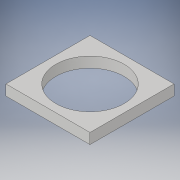
# Autodesk Inventor part: MarbleRingTest3
Saved by Autodesk Inventor 2018 (Build 220112000, 112)
## iProperties
Created: 2019-03-20
Part Number: MarbleRingTest3
Material: Generic
Document SubType Name: Modeling
Designer: 871357
Density: 1 g/cm^3
Appearance: Default
Author: 871357
Autodesk Inventor part; units mm, degrees
ref_plane "YZ Plane" through (0, 0, 0) normal (1, 0, 0) x (0, 1, 0)
ref_plane "XZ Plane" through (0, 0, 0) normal (0, 1, 0) x (-1, 0, 0)
ref_plane "XY Plane" through (0, 0, 0) normal (0, 0, 1) x (1, 0, 0)
sketch "Sketch1" plane through (0, 0, 0) normal (0, 1, 0) x (-1, 0, 0)
  circle A0 centre (0, 0) radius 8.255
  line L0 (10.16, -10.16) -> (-10.16, -10.16)
  line L1 (-10.16, -10.16) -> (-10.16, 10.16)
  line L2 (-10.16, 10.16) -> (10.16, 10.16)
  line L3 (10.16, 10.16) -> (10.16, -10.16)
  dimension "d0" = 16.51
  dimension "d4" = 20.32
  dimension "d5" = 10.16
  dimension "d6" = 20.32
  dimension "d7" = 10.16
  constraints: 8 end point, 2 parallel, 1 centre point, 1 coincident, 1 horizontal, 1 perpendicular
  measures "d0" diameter of A0
  measures "d4" distance between parallel lines of L2 L0
  measures "d5" distance from line of point (0, 0) L0
  measures "d6" distance between parallel lines of L1 L3
  measures "d7" distance from line of point (0, 0) L1
extrude "Extrusion2" add sketch "Sketch1" along normal blind 2.54
body "Solid2"
